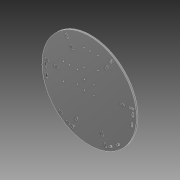
# Autodesk Inventor part: Основание_нижнее
Saved by Autodesk Inventor 2022 (Build 260153000, 153)
## iProperties
Created: 2025-01-10
Part Number: Основание_нижнее
Material: Типовые
Document SubType Name: Modeling
Designer: Ivan
Density: 1 g/cm^3
Appearance: Гладкий — нейтральный серый
Mass: 599.25 g
Surface Area: 2124.2 cm^2
Volume: 599.25 cm^3
Author: Ivan
Title: Основание_нижнее
Autodesk Inventor part; units mm, degrees
ref_plane "РабПлоскость1" through (46.2502, -49.2877, -184.0056) normal (0, 0, 1) x (0.3827, 0.9239, 0)
sketch "Эскиз1" plane through (46.2502, -49.2877, -184.0056) normal (0, 0, 1) x (0.3827, 0.9239, 0)
  arc A0 (-6.0083, -38.3575) -> (120.8555, -172.4727) centre (169.686, 0.7774) ccw construction
  circle A1 centre (169.686, 0.7774) radius 180
  line L0 (16.5638, -6.2333) -> (16.4068, -0.2354) projected
  line L1 (1.4119, -0.628) -> (16.4068, -0.2354) projected
  line L2 (1.569, -6.626) -> (1.4119, -0.628) projected
  line L3 (16.5638, -6.2333) -> (1.569, -6.626) projected
  line L4 (51.3948, 0.6808) -> (51.5518, -5.3171) projected
  line L5 (36.3999, 0.2882) -> (51.3948, 0.6808) projected
  line L6 (36.557, -5.7098) -> (36.3999, 0.2882) projected
  line L7 (51.5518, -5.3171) -> (36.557, -5.7098) projected
  line L8 (136.419, -150.6403) -> (130.5848, -149.2396) projected
  line L9 (127.0831, -163.8252) -> (130.5848, -149.2396) projected
  line L10 (132.9173, -165.2259) -> (127.0831, -163.8252) projected
  line L11 (136.419, -150.6403) -> (132.9173, -165.2259) projected
  line L12 (138.7554, -115.2067) -> (144.5896, -116.6074) projected
  line L13 (135.2537, -129.7922) -> (138.7554, -115.2067) projected
  line L14 (141.0879, -131.1929) -> (135.2537, -129.7922) projected
  line L15 (144.5896, -116.6074) -> (141.0879, -131.1929) projected
  line L16 (240.2947, -96.2969) -> (245.0571, -92.6474) projected
  line L17 (249.4184, -108.2031) -> (240.2947, -96.2969) projected
  line L18 (254.1809, -104.5536) -> (249.4184, -108.2031) projected
  line L19 (245.0571, -92.6474) -> (254.1809, -104.5536) projected
  line L20 (266.3459, -120.4285) -> (261.5834, -124.078) projected
  line L21 (270.7071, -135.9842) -> (261.5834, -124.078) projected
  line L22 (275.4696, -132.3347) -> (270.7071, -135.9842) projected
  line L23 (266.3459, -120.4285) -> (275.4696, -132.3347) projected
  line L24 (257.5837, 24.1469) -> (256.2302, 29.9922) projected
  line L25 (241.6169, 26.6085) -> (256.2302, 29.9922) projected
  line L26 (242.9703, 20.7632) -> (241.6169, 26.6085) projected
  line L27 (257.5837, 24.1469) -> (242.9703, 20.7632) projected
  line L28 (290.3281, 37.8875) -> (291.6816, 32.0422) projected
  line L29 (275.7147, 34.5038) -> (290.3281, 37.8875) projected
  line L30 (277.0682, 28.6585) -> (275.7147, 34.5038) projected
  line L31 (291.6816, 32.0422) -> (277.0682, 28.6585) projected
  line L32 (229.5815, 104.8039) -> (224.3086, 107.6669) projected
  line L33 (236.7388, 117.9862) -> (229.5815, 104.8039) projected
  line L34 (231.4659, 120.8491) -> (236.7388, 117.9862) projected
  line L35 (224.3086, 107.6669) -> (231.4659, 120.8491) projected
  line L36 (241.0091, 138.4255) -> (246.282, 135.5625) projected
  line L37 (253.4394, 148.7448) -> (246.282, 135.5625) projected
  line L38 (248.1665, 151.6077) -> (253.4394, 148.7448) projected
  line L39 (241.0091, 138.4255) -> (248.1665, 151.6077) projected
  line L40 (52.83, 82.5251) -> (48.8152, 78.0662) projected
  line L41 (59.9624, 68.0293) -> (48.8152, 78.0662) projected
  line L42 (63.9772, 72.4881) -> (59.9624, 68.0293) projected
  line L43 (52.83, 82.5251) -> (63.9772, 72.4881) projected
  line L44 (22.8052, 101.4858) -> (26.8199, 105.9447) projected
  line L45 (33.9523, 91.4489) -> (22.8052, 101.4858) projected
  line L46 (37.9671, 95.9077) -> (33.9523, 91.4489) projected
  line L47 (26.8199, 105.9447) -> (37.9671, 95.9077) projected
  point P0 (27.8367, 61.5912)
  constraints: 1 coincident, 3 other
extrude "Выдавливание1" add sketch "Эскиз1" along normal blind 6 contours A1 | L3 L2 L1 L0 | L4 L7 L6 L5 | L11 L10 L9 L8 | L12 L15 L14 L13 | L16 L19 L18 L17 | L23 L22 L21 L20 | L27 L26 L25 L24 | L28 L31 L30 L29 | L32 L35 L34 L33 | L39 L38 L37 L36 | L43 L42 L41 L40 | L44 L47 L46 L45
sketch "Эскиз2" plane through (110.4681, 107.7791, -178.0056) normal (0, 0, 1) x (1, 0, 0)
  line L0 (119.365, 12.6888) -> (118.5818, 18.6375) projected
  line L1 (134.2366, 14.6467) -> (119.365, 12.6888) projected
  line L2 (133.4535, 20.5954) -> (134.2366, 14.6467) projected
  line L3 (118.5818, 18.6375) -> (133.4535, 20.5954) projected
  line L4 (153.2824, 23.2059) -> (154.0655, 17.2572) projected
  line L5 (168.9372, 19.2151) -> (154.0655, 17.2572) projected
  line L6 (168.154, 25.1638) -> (168.9372, 19.2151) projected
  line L7 (153.2824, 23.2059) -> (168.154, 25.1638) projected
  line L8 (65.3227, 100.7072) -> (60.2089, 103.8455) projected
  line L9 (73.1685, 113.4918) -> (65.3227, 100.7072) projected
  line L10 (68.0546, 116.63) -> (73.1685, 113.4918) projected
  line L11 (60.2089, 103.8455) -> (68.0546, 116.63) projected
  line L12 (78.5156, 133.6761) -> (83.6294, 130.5378) projected
  line L13 (91.4751, 143.3224) -> (83.6294, 130.5378) projected
  line L14 (86.3613, 146.4606) -> (91.4751, 143.3224) projected
  line L15 (78.5156, 133.6761) -> (86.3613, 146.4606) projected
  line L16 (-118.5818, 18.6375) -> (-119.365, 12.6888) projected
  line L17 (-133.4535, 20.5954) -> (-118.5818, 18.6375) projected
  line L18 (-134.2366, 14.6467) -> (-133.4535, 20.5954) projected
  line L19 (-119.365, 12.6888) -> (-134.2366, 14.6467) projected
  line L20 (-154.0655, 17.2572) -> (-153.2824, 23.2059) projected
  line L21 (-168.154, 25.1638) -> (-153.2824, 23.2059) projected
  line L22 (-168.9372, 19.2151) -> (-168.154, 25.1638) projected
  line L23 (-154.0655, 17.2572) -> (-168.9372, 19.2151) projected
  line L24 (-56.5443, -144.3494) -> (-62.0876, -142.0533) projected
  line L25 (-67.8278, -155.9115) -> (-62.0876, -142.0533) projected
  line L26 (-62.2845, -158.2076) -> (-67.8278, -155.9115) projected
  line L27 (-56.5443, -144.3494) -> (-62.2845, -158.2076) projected
  line L28 (-48.6937, -109.7175) -> (-43.1504, -112.0136) projected
  line L29 (-54.4339, -123.5757) -> (-48.6937, -109.7175) projected
  line L30 (-48.8906, -125.8718) -> (-54.4339, -123.5757) projected
  line L31 (-43.1504, -112.0136) -> (-48.8906, -125.8718) projected
  line L32 (62.0876, -142.0533) -> (56.5443, -144.3494) projected
  line L33 (62.2845, -158.2076) -> (56.5443, -144.3494) projected
  line L34 (67.8278, -155.9115) -> (62.2845, -158.2076) projected
  line L35 (62.0876, -142.0533) -> (67.8278, -155.9115) projected
  line L36 (43.1504, -112.0136) -> (48.6937, -109.7175) projected
  line L37 (48.8906, -125.8718) -> (43.1504, -112.0136) projected
  line L38 (54.4339, -123.5757) -> (48.8906, -125.8718) projected
  line L39 (48.6937, -109.7175) -> (54.4339, -123.5757) projected
  line L40 (-83.6294, 130.5378) -> (-78.5156, 133.6761) projected
  line L41 (-86.3613, 146.4606) -> (-78.5156, 133.6761) projected
  line L42 (-91.4751, 143.3224) -> (-86.3613, 146.4606) projected
  line L43 (-83.6294, 130.5378) -> (-91.4751, 143.3224) projected
  line L44 (-60.2089, 103.8455) -> (-65.3227, 100.7072) projected
  line L45 (-68.0546, 116.63) -> (-60.2089, 103.8455) projected
  line L46 (-73.1685, 113.4918) -> (-68.0546, 116.63) projected
  line L47 (-65.3227, 100.7072) -> (-73.1685, 113.4918) projected
  point P0 (-110.4681, -107.7791)
extrude "Выдавливание2" cut sketch "Эскиз2" against normal through all
sketch "Эскиз3" plane through (110.4681, 107.7791, -178.0056) normal (0, 0, 1) x (1, 0, 0)
  line L0 (163.5624, 10.7856) -> (169.5396, 10.2627) projected
  line L1 (162.2551, -4.1573) -> (163.5624, 10.7856) projected
  line L2 (168.2323, -4.6802) -> (162.2551, -4.1573) projected
  line L3 (169.5396, 10.2627) -> (168.2323, -4.6802) projected
  line L4 (166.4892, -24.6041) -> (160.512, -24.0812) projected
  line L5 (159.2046, -39.0241) -> (160.512, -24.0812) projected
  line L6 (165.1818, -39.547) -> (159.2046, -39.0241) projected
  line L7 (166.4892, -24.6041) -> (165.1818, -39.547) projected
  line L8 (113.3982, -118.3632) -> (116.8396, -123.2781) projected
  line L9 (101.1109, -126.9669) -> (113.3982, -118.3632) projected
  line L10 (104.5524, -131.8818) -> (101.1109, -126.9669) projected
  line L11 (116.8396, -123.2781) -> (104.5524, -131.8818) projected
  line L12 (88.1693, -143.3533) -> (84.7279, -138.4384) projected
  line L13 (72.4406, -147.042) -> (84.7279, -138.4384) projected
  line L14 (75.882, -151.957) -> (72.4406, -147.042) projected
  line L15 (88.1693, -143.3533) -> (75.882, -151.957) projected
  line L16 (-169.5396, 10.2627) -> (-163.5624, 10.7856) projected
  line L17 (-168.2323, -4.6802) -> (-169.5396, 10.2627) projected
  line L18 (-162.2551, -4.1573) -> (-168.2323, -4.6802) projected
  line L19 (-163.5624, 10.7856) -> (-162.2551, -4.1573) projected
  line L20 (-160.512, -24.0812) -> (-166.4892, -24.6041) projected
  line L21 (-165.1818, -39.547) -> (-166.4892, -24.6041) projected
  line L22 (-159.2046, -39.0241) -> (-165.1818, -39.547) projected
  line L23 (-160.512, -24.0812) -> (-159.2046, -39.0241) projected
  line L24 (-116.8396, -123.2781) -> (-113.3982, -118.3632) projected
  line L25 (-104.5524, -131.8818) -> (-116.8396, -123.2781) projected
  line L26 (-101.1109, -126.9669) -> (-104.5524, -131.8818) projected
  line L27 (-113.3982, -118.3632) -> (-101.1109, -126.9669) projected
  line L28 (-84.7279, -138.4384) -> (-88.1693, -143.3533) projected
  line L29 (-75.882, -151.957) -> (-88.1693, -143.3533) projected
  line L30 (-72.4406, -147.042) -> (-75.882, -151.957) projected
  line L31 (-84.7279, -138.4384) -> (-72.4406, -147.042) projected
  point P0 (-110.4681, -107.7791)
extrude "Выдавливание3" cut sketch "Эскиз3" against normal through all
sketch "Эскиз4" plane through (110.4681, 107.7791, -184.0056) normal (0, 0, -1) x (-1, 0, 0)
  circle A0 centre (0, 0) radius 180 construction
  circle A1 centre (0, 0) radius 180 construction
  line L0 (200, -150) -> (-200, -150)
  line L1 (-200, -150) -> (-200, 150)
  line L2 (-200, 150) -> (200, 150)
  line L3 (200, 150) -> (200, -150)
  line L4 (200, -150) -> (-200, 150) construction
  line L5 (-200, -150) -> (200, 150) construction
  line L6 (-262.6084, 185.8696) -> (306.1084, 185.8696)
  line L7 (306.1084, 185.8696) -> (306.1084, -212.6524)
  line L8 (306.1084, -212.6524) -> (-262.6084, -212.6524)
  line L9 (-262.6084, -212.6524) -> (-262.6084, 185.8696)
  point P0 (110.4681, -107.7791)
  dimension "d6" = 400
  dimension "d7" = 300
  constraints: 20 end point, 4 parallel, 2 horizontal, 2 midpoint, 2 perpendicular
  measures "d6" distance of L1.end L2.end
  measures "d7" distance of L2.end L0.start
extrude "Выдавливание4" [suppressed]
sketch "Эскиз5" plane through (46.2502, -49.2877, -184.0056) normal (0, 0, -1) x (-0.9239, 0.3827, 0)
  arc A0 (32.2974, 186.9869) -> (-9.2771, 204.2076) centre (4.5085, 178.6938) ccw construction
  line L0 (32.2974, 186.9869) -> (18.2942, 153.1799) construction
  arc A1 (-23.2804, 170.4007) -> (18.2942, 153.1799) centre (4.5085, 178.6938) ccw construction
  line L1 (-23.2804, 170.4007) -> (-9.2771, 204.2076) construction
  circle A2 centre (-0.1125, 153.8187) radius 1.6 construction
  circle A3 centre (-9.8133, 157.8368) radius 1.6 construction
  circle A4 centre (18.8303, 199.5507) radius 1.6 construction
  circle A5 centre (9.1296, 203.5689) radius 1.6 construction
  circle A6 centre (-18.5885, 169.1267) radius 1.6 construction
  circle A7 centre (-5.0586, 201.7908) radius 1.6 construction
  circle A8 centre (27.6055, 188.2609) radius 1.6 construction
  circle A9 centre (14.0756, 155.5968) radius 1.6 construction
  line L2 (5.8066, 155.6964) -> (21.688, 194.0374) construction
  line L3 (21.688, 194.0374) -> (15.2208, 196.7162) construction
  line L4 (15.2208, 196.7162) -> (15.9862, 198.564) construction
  arc A10 (15.9862, 198.564) -> (10.4429, 200.8601) centre (12.8797, 198.9036) ccw construction
  line L5 (10.4429, 200.8601) -> (9.6776, 199.0123) construction
  line L6 (9.6776, 199.0123) -> (3.2104, 201.6911) construction
  line L7 (3.2104, 201.6911) -> (-12.671, 163.3501) construction
  line L8 (-12.671, 163.3501) -> (-6.2038, 160.6713) construction
  line L9 (-6.2038, 160.6713) -> (-6.9692, 158.8236) construction
  arc A11 (-6.9692, 158.8236) -> (-1.4259, 156.5275) centre (-3.8627, 158.4839) ccw construction
  line L10 (-1.4259, 156.5275) -> (-0.6605, 158.3752) construction
  line L11 (-0.6605, 158.3752) -> (5.8066, 155.6964) construction
  point P0 (61.5912, 27.8367)
  constraints: 4 coincident
hole "Отверстие1" at (92.7904, 99.8515, -184.0056) at (92.7904, 135.2068, -184.0056) at (128.1457, 135.2068, -184.0056) at (128.1457, 99.8515, -184.0056) direction (0, 0, 1) diameter 3.2 end through all clearance for "болты с шестигранной головкой / гайка ГОСТ 12876-67" size "M3" standard "ГОСТ"
sketch "Эскиз6" plane through (46.2502, -49.2877, -184.0056) normal (0, 0, -1) x (-0.9239, 0.3827, 0)
  circle A0 centre (84.4983, 114.7398) radius 1.625 construction
  circle A1 centre (41.5968, 150.3155) radius 1.625 construction
  circle A2 centre (60.4057, 195.7242) radius 1.625 construction
  circle A3 centre (88.6061, 184.1055) radius 1.625 construction
  circle A4 centre (109.4096, 175.5344) radius 1.625 construction
  point P0 (61.5912, 27.8367)
  constraints: 5 coincident
hole "Отверстие2" at (12.0931, 89.0541, -184.0056) at (65.3431, 105.5041, -184.0056) at (12.3431, 154.7541, -184.0056) at (34.8431, 154.7117, -184.0056) at (65.3431, 154.6541, -184.0056) direction (0, 0, 1) diameter 3.2 end through all clearance for "болты с шестигранной головкой / гайка ГОСТ 12876-67" size "M3" standard "ГОСТ"
sketch "Эскиз7" plane through (46.2502, -49.2877, -184.0056) normal (0, 0, -1) x (-0.9239, 0.3827, 0)
  point P0 (61.5912, 27.8367)
  point P1 (44.478, 223.3708)
  point P2 (1.5454, 258.9374)
  point P3 (20.3051, 304.1993)
  point P4 (48.5237, 292.5107)
  point P5 (69.3361, 283.9798)
hole "Отверстие3" at (90.6382, 174.101, -184.0056) at (143.9136, 190.5306, -184.0056) at (143.9028, 239.5262, -184.0056) at (113.3591, 239.5262, -184.0056) at (90.8664, 239.6092, -184.0056) direction (0, 0, 1) diameter 3.2 end through all clearance for "болты с шестигранной головкой / гайка ГОСТ 12876-67" size "M3" standard "ГОСТ"
sketch "Эскиз8" plane through (110.4681, 107.7791, -178.0056) normal (0, 0, 1) x (1, 0, 0)
  circle A0 centre (0, 0) radius 180 construction
  line L0 (0, 0) -> (0, 208.8659)
  line L1 (0, 0) -> (227.021, 0)
  point P0 (-110.4681, -107.7791)
  constraints: 4 end point, 1 horizontal, 1 vertical
ref_plane "РабПлоскость2" through (110.4681, 107.7791, -178.0056) normal (1, 0, 0) x (0, 1, 0)
ref_plane "РабПлоскость3" through (110.4681, 107.7791, -178.0056) normal (0, 1, 0) x (-1, 0, 0)
